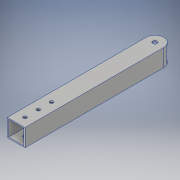
# Autodesk Inventor part: CLB_036_FourPartScissorBarTop
Saved by Autodesk Inventor 2018.3 (Build 223284000, 284)
## iProperties
Created: 2020-01-12
Part Number: CLB_036_FourPartScissorBarTop
Material: Aluminum 6061
Document SubType Name: Modeling
Designer: Cooper
Density: 2.7 g/cm^3
Appearance: Aluminum - Flat
Mass: 227.288 g
Surface Area: 1065.51 cm^2
Volume: 84.1809 cm^3
Author: Cooper
Autodesk Inventor part; units mm, degrees
ref_plane "YZ Plane" through (0, 0, 0) normal (1, 0, 0) x (0, 1, 0)
ref_plane "XZ Plane" through (0, 0, 0) normal (0, 1, 0) x (-1, 0, 0)
ref_plane "XY Plane" through (0, 0, 0) normal (0, 0, 1) x (1, 0, 0)
sketch "Sketch1" plane through (0, 0, 0) normal (0, 0, 1) x (1, 0, 0)
  line L0 (0, 0) -> (25.4, 0)
  line L1 (25.4, 0) -> (25.4, 25.4)
  line L2 (25.4, 25.4) -> (0, 25.4)
  line L3 (0, 25.4) -> (0, 0)
  line L4 (1.5875, 1.5875) -> (23.8125, 1.5875)
  line L5 (23.8125, 1.5875) -> (23.8125, 23.8125)
  line L6 (23.8125, 23.8125) -> (1.5875, 23.8125)
  line L7 (1.5875, 23.8125) -> (1.5875, 1.5875)
  dimension "d0" = 25.4
  dimension "d1" = 25.4
  dimension "d2" = 1.5875
  constraints: 16 end point, 4 parallel, 2 perpendicular, 1 horizontal, 3 other
  measures "d0" distance of L2.end L0.start
  measures "d1" distance of L0.start L0.end
  measures "d2" distance between parallel lines of L6 L2
extrude "Extrusion1" add sketch "Sketch1" along normal blind 400.05
sketch "Sketch3" plane through (0, 25.4, 0) normal (0, 1, 0) x (1, 0, 0)
  line L0 (25.4, 0) -> (0, 0) projected
  line L1 (0, 0) -> (0, -400.05) projected
  line L2 (25.4, -400.05) -> (0, -400.05) projected
  line L3 (25.4, 0) -> (25.4, -400.05) projected
  point P0 (0, 0)
  point P1 (12.7, -200.025)
  dimension "d15" = 200.025
  dimension "d16" = 400.05
  dimension "d17" = 12.7
  measures "d15" distance from line of point (12.7, -200.025) L2
  measures "d16" distance between parallel lines of L0 L2
  measures "d17" distance from line of L1 point (12.7, -200.025)
hole "Hole2" at (12.7, 25.4, 200.025) direction (0, -1, 0) diameter 6.35 end through all clearance for "Flat Head Machine Screw (82)" size "1/4" standard "Ansi Unified Screw Threads"
sketch "Sketch7" plane through (0, 25.4, 0) normal (0, 1, 0) x (1, 0, 0)
  line L0 (0, 0) -> (0, -400.05) projected
  line L1 (25.4, 0) -> (25.4, -400.05) projected
  line L2 (25.4, 0) -> (0, 0) projected
  line L3 (0, 0) -> (25.4, 0) projected
  line L4 (0, -200.025) -> (0, 0)
  line L5 (25.4, 0) -> (25.4, -200.025)
  line L6 (0, 0) -> (25.4, 0)
  arc A0 (25.4, -200.025) -> (0, -200.025) centre (12.7, -200.025) ccw
  line L7 (25.4, -400.05) -> (0, -400.05) projected
  circle A1 centre (12.7, -200.025) radius 3.175 projected
  line L8 (25.4, 0) -> (0, 0) projected
  line L9 (0, 0) -> (0, -400.05) projected
  line L10 (25.4, -400.05) -> (0, -400.05) projected
  line L11 (25.4, 0) -> (25.4, -400.05) projected
  constraints: 6 end point, 2 midpoint, 2 point on circle, 2 tangent, 1 centre point, 1 coincident, 1 collinear, 1 perpendicular
extrude "Extrusion3" cut sketch "Sketch7" against normal blind 25.4 contours L2 L1 A0 L0
sketch "Sketch8" plane through (0, 25.4, 400.05) normal (0, 1, 0) x (1, 0, 0)
  line L0 (25.4, 0) -> (0, 0) projected
  line L1 (0, 200.025) -> (0, 0) projected
  point P0 (0, 400.05)
  point P1 (12.7, 12.7)
  point P2 (12.7, 31.75)
  point P3 (12.7, 50.8)
  dimension "d43" = 12.7
  dimension "d44" = 12.7
  dimension "d55" = 19.05
  dimension "d56" = 19.05
  constraints: 2 vertical alignment
  measures "d43" distance from line of L0 point (12.7, 12.7)
  measures "d44" distance from line of L1 point (12.7, 12.7)
  measures "d55" distance of point (12.7, 31.75) point (12.7, 12.7)
  measures "d56" distance of point (12.7, 50.8) point (12.7, 31.75)
hole "Hole4" at (12.7, 25.4, 387.35) at (12.7, 25.4, 368.3) at (12.7, 25.4, 349.25) direction (0, -1, 0) diameter 4.8514 end through all
equation "\"d15\" = 0.5 * d16"
body "Solid1"
